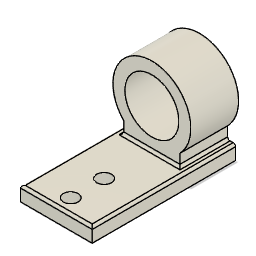
Flow+Sensor+Mount (Autodesk Fusion 360 design; units mm, degrees)
Autodesk Fusion 360 part; units mm, degrees
sketch "Sketch1" plane through (0, 0, 0) normal (0, 0, 1) x (1, 0, 0)
  line L0 (0, 0) -> (15, 0)
  line L1 (15, 0) -> (15, 3)
  line L2 (15, 3) -> (0, 3)
  line L3 (0, 3) -> (0, 0)
  line L4 (1.6263, 3) -> (13.3737, 3)
  line L5 (13.3737, 3) -> (13.3737, 5.5)
  line L6 (13.3737, 5.5) -> (1.6263, 5.5)
  line L7 (1.6263, 5.5) -> (1.6263, 3)
  circle A0 centre (7.5, 11.15) radius 8.15
  circle A1 centre (7.5, 11.15) radius 5.65
  line L8 (7.5, 0) -> (7.5, 3) construction
  line L9 (7.5, 5.5) -> (7.5, 3) construction
  dimension "d1" = 11.3
  dimension "d2" = 15
  dimension "d4" = 3
  dimension "d19" = 2.5
  constraint horizontal L0
  constraint vertical L1
  constraint horizontal L2
  constraint vertical L3
  constraint coincident L0.start L3.end
  constraint horizontal L4
  constraint vertical L5
  constraint horizontal L6
  constraint vertical L7
  constraint coincident L2 L4.start
  constraint concentric A0 A1
  constraint tangent L4 A0
  constraint tangent L6 A1
  constraint midpoint L0 L8.start
  constraint midpoint L2 L8.end
  constraint midpoint L6 L9.start
  constraint midpoint L4 L8.end
  constraint collinear L8 L9
  constraint coincident A1 L9.start
  constraint coincident L5.end A0
  measures "d1" diameter of A1
  measures "d2" distance of L0.start L0.end
  measures "d4" distance of L0.end L1.end
  measures "d19" distance of A0 A1
extrude "Extrude1" add sketch "Sketch1" along normal blind 10 contours L2 L4 L7 A0 | L2 L4 L5 A0 | L6 A0 | L6 A0
extrude "Extrude2" add sketch "Sketch1" along normal blind 30 contours L0 L1 L2 L3 L4
sketch "Sketch2" plane through (0, 3, 0) normal (0, 1, 0) x (-1, 0, 0)
  line L0 (-13.3737, 0) -> (-13.3737, 10)
  line L1 (-13.3737, 10) -> (-1.6263, 10)
  line L2 (-1.6263, 10) -> (-1.6263, 0)
  line L3 (-1.6263, 0) -> (0, 0)
  line L4 (0, 0) -> (0, 30)
  line L5 (0, 30) -> (-15, 30)
  line L6 (-15, 30) -> (-15, 0)
  line L7 (-15, 0) -> (-13.3737, 0)
  line L8 (-7.5, 30) -> (-7.5, 10) construction
  circle A0 centre (-7.5, 27) radius 1.55
  circle A1 centre (-7.5, 20) radius 1.55
  dimension "d9" = 3.1
  dimension "d10" = 3.1
  dimension "d11" = 7
  dimension "d12" = 3
  constraint midpoint L5 L8.start
  constraint midpoint L1 L8.end
  constraint coincident L8 A0.centre
  constraint coincident L8 A1.centre
  measures "d9" diameter of A0
  measures "d10" diameter of A1
  measures "d11" distance of A0.centre A1.centre
  measures "d12" distance of L5 A0.centre
extrude "Extrude3" cut sketch "Sketch2" against normal up to surface (3 mm away) contours A0 | A1
fillet "Fillet1" radius 0.5 3 edges at (0, 3, 15) (7.5, 3, 30) (15, 3, 15)
fillet "Fillet2" radius 0.5 3 edges at (13.3737, 3, 5) (7.5, 3, 10) (1.6263, 3, 5)
equation "d10 = d9"
